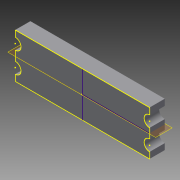
# Autodesk Inventor part: bottom_pcb
Saved by Autodesk Inventor 2014 (Build 180170000, 170)
## iProperties
Created: 2013-06-27
Part Number: bottom_pcb
Material: Generisch
Document SubType Name: Modeling
Designer: hanse
Density: 1 g/cm^3
Appearance: Vorgabe
Mass: 0.0128956 g
Surface Area: 0.48455 cm^2
Volume: 0.0128956 cm^3
Author: hanse
Autodesk Inventor part; units mm, degrees
ref_plane "YZ Plane" through (0, 0, 0) normal (1, 0, 0) x (0, 1, 0)
ref_plane "XZ Plane" through (0, 0, 0) normal (0, 1, 0) x (-1, 0, 0)
ref_plane "XY Plane" through (0, 0, 0) normal (0, 0, 1) x (1, 0, 0)
sketch "Skizze1" plane through (0, 0, 0) normal (0, 1, 0) x (-1, 0, 0)
  line L0 (0, 0) -> (7.1, 0)
  line L1 (7.1, 0) -> (7.1, 2.35)
  line L2 (7.1, 2.35) -> (0, 2.35)
  line L3 (0, 2.35) -> (0, 0)
  dimension "d0" = 7.1
  dimension "d1" = 2.35
  constraints: 8 end point, 2 parallel, 1 horizontal, 1 perpendicular
  measures "d0" distance of L2.end L1.end
  measures "d1" distance of L1.end L0.end
extrude "Extrusion1" add sketch "Skizze1" along normal blind 0.8
sketch "Skizze2" plane through (0, 0.8, 0) normal (0, 1, 0) x (1, 0, 0)
  line L0 (0, 0) -> (-7.1, 0) projected
  line L1 (-7.1, 0) -> (-7.1, -2.35) projected
  line L2 (0, -2.35) -> (0, 0) projected
  circle A0 centre (0, -0.62) radius 0.3
  circle A1 centre (0, -1.72) radius 0.3
  circle A2 centre (-7.1, -0.625) radius 0.3
  circle A3 centre (-7.1, -1.725) radius 0.3
  dimension "d4" = 0.6
  dimension "d5" = 0.6
  dimension "d6" = 0.6
  dimension "d7" = 0.6
  dimension "d8" = 1.1
  dimension "d9" = 1.1
  dimension "d10" = 0.625
  dimension "d11" = 0.62
  constraints: 4 centre point, 4 point on line
  measures "d4" diameter of A0
  measures "d5" diameter of A1
  measures "d6" diameter of A2
  measures "d7" diameter of A3
  measures "d8" distance of A3.centre A2.centre
  measures "d9" distance of A1.centre A0.centre
  measures "d10" distance from line of L0 A2.centre
  measures "d11" distance of L0.start A0.centre
extrude "Extrusion2" cut sketch "Skizze2" against normal through all
sketch "Skizze3" plane through (0, 0, 0) normal (0, -1, 0) x (1, 0, 0)
  arc A0 (-7.1, 1.425) -> (-7.1, 2.025) centre (-7.1, 1.725) ccw projected
  line L0 (-7.1, 0.925) -> (-7.1, 1.425) projected
  arc A1 (-7.1, 0.325) -> (-7.1, 0.925) centre (-7.1, 0.625) ccw projected
  line L1 (-7.1, 0) -> (-7.1, 0.325) projected
  line L2 (0, 0) -> (-7.1, 0) projected
  line L3 (0, 0.32) -> (0, 0) projected
  arc A2 (0, 0.92) -> (0, 0.32) centre (0, 0.62) ccw projected
  line L4 (0, 1.42) -> (0, 0.92) projected
  arc A3 (0, 2.02) -> (0, 1.42) centre (0, 1.72) ccw projected
  line L5 (0, 2.35) -> (0, 2.02) projected
  line L6 (-7.1, 2.35) -> (0, 2.35) projected
  line L7 (-7.1, 2.025) -> (-7.1, 2.35) projected
  line L8 (-3.55, 2.35) -> (-3.55, 0)
  line L9 (-3.55, 1.175) -> (0, 1.17)
  constraints: 4 end point, 4 midpoint
ref_plane "Arbeitsebene1" through (-3.55, 0, 1.175) normal (0, 0, 1) x (1, 0, 0)
